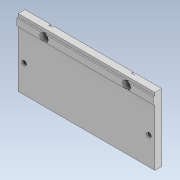
# Autodesk Inventor part: Klipper_Expander_Mount
Saved by Autodesk Inventor 2022.1 (Build 261234020, 234B)
## iProperties
Created: 2022-07-30
Part Number: Klipper_Expander_Mount
Material: Generisch
Document SubType Name: Modeling
Designer: Rama
Density: 1 g/cm^3
Appearance: Vorgabe
Author: Rama
Autodesk Inventor part; units mm, degrees
ref_plane "YZ Plane" through (0, 0, 0) normal (1, 0, 0) x (0, 1, 0)
ref_plane "XZ Plane" through (0, 0, 0) normal (0, 1, 0) x (-1, 0, 0)
ref_plane "XY Plane" through (0, 0, 0) normal (0, 0, 1) x (1, 0, 0)
sketch "Skizze1" plane through (0, 0, 0) normal (0, 0, 1) x (1, 0, 0)
  line L0 (50, -12) -> (-50, -12) projected
  line L1 (50, 12) -> (50, -12) projected
  line L2 (-50, 12) -> (50, 12) projected
  line L3 (-50, -12) -> (-50, 12) projected
  circle A0 centre (-21.494, -8.778) radius 0.5 projected
  circle A1 centre (-18.954, -8.778) radius 0.5 projected
  circle A2 centre (-13.874, -8.778) radius 0.5 projected
  circle A3 centre (-16.414, -8.778) radius 0.5 projected
  circle A4 centre (-3, 1.025) radius 0.85 projected
  circle A5 centre (-3, -2.635) radius 0.85 projected
  circle A6 centre (-1.67, -8.75) radius 0.5 projected
  circle A7 centre (-4.21, -8.75) radius 0.5 projected
  circle A8 centre (-6.75, -8.75) radius 0.5 projected
  circle A9 centre (-14.35, 5.5) radius 0.65 projected
  circle A10 centre (-9.27, 5.5) radius 0.65 projected
  circle A11 centre (-3, 5.495) radius 0.85 projected
  circle A12 centre (13.41, 5.5) radius 0.65 projected
  circle A13 centre (10.31, -9.613) radius 0.625 projected
  circle A14 centre (8.33, 5.5) radius 0.65 projected
  circle A15 centre (3.25, 5.5) radius 0.65 projected
  circle A16 centre (3.81, -9.613) radius 0.625 projected
  circle A17 centre (-26.341, -8.851) radius 0.5 projected
  circle A18 centre (-26.341, -6.311) radius 0.5 projected
  circle A19 centre (-26.341, -3.771) radius 0.5 projected
  circle A20 centre (-47.25, 1.58) radius 0.5 projected
  circle A21 centre (-47.25, -0.96) radius 0.5 projected
  circle A22 centre (-47.25, -3.5) radius 0.5 projected
  circle A23 centre (-41.75, -7.5) radius 0.5 projected
  circle A24 centre (-41.75, -4.96) radius 0.5 projected
  circle A25 centre (-47.25, -8.5) radius 0.5 projected
  circle A26 centre (-33, -4.96) radius 0.5 projected
  circle A27 centre (-33, -7.5) radius 0.5 projected
  circle A28 centre (-3, 9.155) radius 0.85 projected
  circle A29 centre (-34.242, 7.8785) radius 0.425 projected
  circle A30 centre (-29.242, 7.8785) radius 0.425 projected
  circle A31 centre (-22.54, 9) radius 0.5 projected
  circle A32 centre (-20, 9) radius 0.5 projected
  line L4 (-27.942, 10.9285) -> (-27.942, 10.2285) projected
  arc A33 (-28.542, 10.2285) -> (-27.942, 10.2285) centre (-28.242, 10.2285) ccw projected
  line L5 (-28.542, 10.2285) -> (-28.542, 10.9285) projected
  arc A34 (-27.942, 10.9285) -> (-28.542, 10.9285) centre (-28.242, 10.9285) ccw projected
  circle A35 centre (-46, 8) radius 1.6 projected
  line L6 (-34.942, 10.9285) -> (-34.942, 10.2285) projected
  arc A36 (-35.542, 10.2285) -> (-34.942, 10.2285) centre (-35.242, 10.2285) ccw projected
  line L7 (-35.542, 10.2285) -> (-35.542, 10.9285) projected
  arc A37 (-34.942, 10.9285) -> (-35.542, 10.9285) centre (-35.242, 10.9285) ccw projected
  circle A38 centre (33.73, 5.5) radius 0.65 projected
  circle A39 centre (28.65, 5.5) radius 0.65 projected
  circle A40 centre (18.49, 5.5) radius 0.65 projected
  circle A41 centre (23.57, 5.5) radius 0.65 projected
  circle A42 centre (38.81, 5.5) radius 0.65 projected
  circle A43 centre (46, 8) radius 1.6 projected
  line L8 (50.4, 12.4) -> (-50.4, 12.4)
  line L9 (-50.4, 12.4) -> (-50.4, -12.4)
  line L10 (-50.4, -12.4) -> (50.4, -12.4)
  line L11 (50.4, -12.4) -> (50.4, 12.4)
  point P0 (0, 0)
  dimension "d0" = 0.4
  dimension "d1" = 0.4
  dimension "d2" = 0.4
  dimension "d3" = 0.4
  constraints: 8 end point, 2 parallel, 1 horizontal, 1 perpendicular
  measures "d0" distance between parallel lines of L1 L11
  measures "d1" distance between parallel lines of L0 L10
  measures "d2" distance between parallel lines of L8 L2
  measures "d3" distance between parallel lines of L3 L9
extrude "Extrusion1" add sketch "Skizze1" along normal blind 6 contours L0 L3 L2 L1 | A0 | A1 | A2 | A3 | A4 | A5 | A6 | A7 | A8 | A9 | A10 | A11 | A12 | A13 | A14 | A15 | A16 | A17 | A18 | A19 | A20 | A21 | A22 | A23 | A24 | A25 | A26 | A27 | A28 | A29 | A30 | A31 | A32 | L4 A33 L5 A34 | A35 | L6 A36 L7 A37 | A38 | A39 | A40 | A41 | A42 | A43 | L11 L10 L9 L8
sketch "Skizze2" plane through (0, 0, 0) normal (0, 0, -1) x (-1, 0, 0)
  circle A0 centre (-46, 8) radius 1.6 projected
  circle A1 centre (46, 8) radius 1.6 projected
  point P0 (0, 0)
hole "Bohrung1" at (46, 8, 0) at (-46, 8, 0) direction (0, 0, 1) diameter 3.34 end through all counterbore diameter 4.7 counterbore depth 5
sketch "Skizze3" plane through (-50.4, 12.4, 0) normal (0, 1, 0) x (1, 0, 0)
  line L0 (100.8, 0) -> (0, 0) projected
  line L1 (0, 0) -> (0, -6) projected
  line L2 (100.8, -6) -> (0, -6) projected
  line L3 (100.8, 0) -> (100.8, -6) projected
  point P0 (50.4, 0)
extrude "Extrusion2" add sketch "Skizze3" along normal blind 25
sketch "Skizze4" plane through (50.4, -12.4, 6) normal (1, 0, 0) x (0, 0, -1)
  line L0 (0, 47.8) -> (-2, 47.8) projected
  line L1 (-2, 41.8) -> (0, 41.8) projected
  line L2 (7.6775, 47.7) -> (-1, 47.7)
  line L3 (-1, 47.7) -> (-1, 41.9)
  line L4 (-1, 41.9) -> (7.6775, 41.9)
  line L5 (7.6775, 41.9) -> (7.6775, 47.7)
  line L6 (0, 0) -> (0, 49.8) projected
  point P0 (6, 12.4)
  point P1 (0, 41.9)
  point P2 (0, 47.7)
  dimension "d15" = 0.1
  dimension "d16" = 0.1
  dimension "d17" = 5.8
  dimension "d18" = 1
  constraints: 8 end point, 2 parallel, 1 horizontal, 1 perpendicular
  measures "d15" distance between parallel lines of L0 L2
  measures "d16" distance between parallel lines of L1 L4
  measures "d17" distance of L4.end L2.start
  measures "d18" distance between parallel lines of L6 L3
extrude "Extrusion3" add sketch "Skizze4" against normal up to surface (100.8 mm away) contours L6 L4 L3 L2
sketch "Skizze6" plane through (0, 0, 0) normal (0, 0, -1) x (-1, 0, 0)
  line L0 (-50, -12) -> (50, -12) projected
  line L1 (-50, 12) -> (-50, -12) projected
  line L2 (50, 12) -> (-50, 12) projected
  line L3 (50, -12) -> (50, 12) projected
  circle A0 centre (21.494, -8.778) radius 0.5 projected
  circle A1 centre (18.954, -8.778) radius 0.5 projected
  circle A2 centre (13.874, -8.778) radius 0.5 projected
  circle A3 centre (16.414, -8.778) radius 0.5 projected
  circle A4 centre (3, 1.025) radius 0.85 projected
  circle A5 centre (3, -2.635) radius 0.85 projected
  circle A6 centre (1.67, -8.75) radius 0.5 projected
  circle A7 centre (4.21, -8.75) radius 0.5 projected
  circle A8 centre (6.75, -8.75) radius 0.5 projected
  circle A9 centre (14.35, 5.5) radius 0.65 projected
  circle A10 centre (9.27, 5.5) radius 0.65 projected
  circle A11 centre (3, 5.495) radius 0.85 projected
  circle A12 centre (-13.41, 5.5) radius 0.65 projected
  circle A13 centre (-10.31, -9.613) radius 0.625 projected
  circle A14 centre (-8.33, 5.5) radius 0.65 projected
  circle A15 centre (-3.25, 5.5) radius 0.65 projected
  circle A16 centre (-3.81, -9.613) radius 0.625 projected
  circle A17 centre (26.341, -8.851) radius 0.5 projected
  circle A18 centre (26.341, -6.311) radius 0.5 projected
  circle A19 centre (26.341, -3.771) radius 0.5 projected
  circle A20 centre (47.25, 1.58) radius 0.5 projected
  circle A21 centre (47.25, -0.96) radius 0.5 projected
  circle A22 centre (47.25, -3.5) radius 0.5 projected
  circle A23 centre (41.75, -7.5) radius 0.5 projected
  circle A24 centre (41.75, -4.96) radius 0.5 projected
  circle A25 centre (47.25, -8.5) radius 0.5 projected
  circle A26 centre (33, -4.96) radius 0.5 projected
  circle A27 centre (33, -7.5) radius 0.5 projected
  circle A28 centre (3, 9.155) radius 0.85 projected
  circle A29 centre (34.242, 7.8785) radius 0.425 projected
  circle A30 centre (29.242, 7.8785) radius 0.425 projected
  circle A31 centre (22.54, 9) radius 0.5 projected
  circle A32 centre (20, 9) radius 0.5 projected
  line L4 (27.942, 10.9285) -> (27.942, 10.2285) projected
  arc A33 (27.942, 10.2285) -> (28.542, 10.2285) centre (28.242, 10.2285) ccw projected
  line L5 (28.542, 10.2285) -> (28.542, 10.9285) projected
  arc A34 (28.542, 10.9285) -> (27.942, 10.9285) centre (28.242, 10.9285) ccw projected
  circle A35 centre (46, 8) radius 1.6 projected
  line L6 (34.942, 10.9285) -> (34.942, 10.2285) projected
  arc A36 (34.942, 10.2285) -> (35.542, 10.2285) centre (35.242, 10.2285) ccw projected
  line L7 (35.542, 10.2285) -> (35.542, 10.9285) projected
  arc A37 (35.542, 10.9285) -> (34.942, 10.9285) centre (35.242, 10.9285) ccw projected
  circle A38 centre (-33.73, 5.5) radius 0.65 projected
  circle A39 centre (-28.65, 5.5) radius 0.65 projected
  circle A40 centre (-18.49, 5.5) radius 0.65 projected
  circle A41 centre (-23.57, 5.5) radius 0.65 projected
  circle A42 centre (-38.81, 5.5) radius 0.65 projected
  circle A43 centre (-46, 8) radius 1.6 projected
  point P0 (0, 0)
hole "Bohrung2" at (38.81, 5.5, 0) at (33.73, 5.5, 0) at (28.65, 5.5, 0) at (23.57, 5.5, 0) at (18.49, 5.5, 0) at (13.41, 5.5, 0) at (8.33, 5.5, 0) at (3.25, 5.5, 0) at (-3, 5.495, 0) at (-3, 9.155, 0) at (-3, 1.025, 0) at (-3, -2.635, 0) at (-9.27, 5.5, 0) at (-14.35, 5.5, 0) direction (0, 0, 1) diameter 2.8 depth 2 tip angle 60
sketch "Skizze7" plane through (0, 0, 0) normal (0, 0, -1) x (-1, 0, 0)
  line L0 (-50, -12) -> (50, -12) projected
  line L1 (-50, 12) -> (-50, -12) projected
  line L2 (50, 12) -> (-50, 12) projected
  line L3 (50, -12) -> (50, 12) projected
  circle A0 centre (21.494, -8.778) radius 0.5 projected
  circle A1 centre (18.954, -8.778) radius 0.5 projected
  circle A2 centre (13.874, -8.778) radius 0.5 projected
  circle A3 centre (16.414, -8.778) radius 0.5 projected
  circle A4 centre (3, 1.025) radius 0.85 projected
  circle A5 centre (3, -2.635) radius 0.85 projected
  circle A6 centre (1.67, -8.75) radius 0.5 projected
  circle A7 centre (4.21, -8.75) radius 0.5 projected
  circle A8 centre (6.75, -8.75) radius 0.5 projected
  circle A9 centre (14.35, 5.5) radius 0.65 projected
  circle A10 centre (9.27, 5.5) radius 0.65 projected
  circle A11 centre (3, 5.495) radius 0.85 projected
  circle A12 centre (-13.41, 5.5) radius 0.65 projected
  circle A13 centre (-10.31, -9.613) radius 0.625 projected
  circle A14 centre (-8.33, 5.5) radius 0.65 projected
  circle A15 centre (-3.25, 5.5) radius 0.65 projected
  circle A16 centre (-3.81, -9.613) radius 0.625 projected
  circle A17 centre (26.341, -8.851) radius 0.5 projected
  circle A18 centre (26.341, -6.311) radius 0.5 projected
  circle A19 centre (26.341, -3.771) radius 0.5 projected
  circle A20 centre (47.25, 1.58) radius 0.5 projected
  circle A21 centre (47.25, -0.96) radius 0.5 projected
  circle A22 centre (47.25, -3.5) radius 0.5 projected
  circle A23 centre (41.75, -7.5) radius 0.5 projected
  circle A24 centre (41.75, -4.96) radius 0.5 projected
  circle A25 centre (47.25, -8.5) radius 0.5 projected
  circle A26 centre (33, -4.96) radius 0.5 projected
  circle A27 centre (33, -7.5) radius 0.5 projected
  circle A28 centre (3, 9.155) radius 0.85 projected
  circle A29 centre (34.242, 7.8785) radius 0.425 projected
  circle A30 centre (29.242, 7.8785) radius 0.425 projected
  circle A31 centre (22.54, 9) radius 0.5 projected
  circle A32 centre (20, 9) radius 0.5 projected
  line L4 (27.942, 10.9285) -> (27.942, 10.2285) projected
  arc A33 (27.942, 10.2285) -> (28.542, 10.2285) centre (28.242, 10.2285) ccw projected
  line L5 (28.542, 10.2285) -> (28.542, 10.9285) projected
  arc A34 (28.542, 10.9285) -> (27.942, 10.9285) centre (28.242, 10.9285) ccw projected
  circle A35 centre (46, 8) radius 1.6 projected
  line L6 (34.942, 10.9285) -> (34.942, 10.2285) projected
  arc A36 (34.942, 10.2285) -> (35.542, 10.2285) centre (35.242, 10.2285) ccw projected
  line L7 (35.542, 10.2285) -> (35.542, 10.9285) projected
  arc A37 (35.542, 10.9285) -> (34.942, 10.9285) centre (35.242, 10.9285) ccw projected
  circle A38 centre (-33.73, 5.5) radius 0.65 projected
  circle A39 centre (-28.65, 5.5) radius 0.65 projected
  circle A40 centre (-18.49, 5.5) radius 0.65 projected
  circle A41 centre (-23.57, 5.5) radius 0.65 projected
  circle A42 centre (-38.81, 5.5) radius 0.65 projected
  circle A43 centre (-46, 8) radius 1.6 projected
  point P0 (0, 0)
hole "Bohrung3" at (10.31, -9.613, 0) at (3.81, -9.613, 0) at (-1.67, -8.75, 0) at (-4.21, -8.75, 0) at (-6.75, -8.75, 0) at (-13.874, -8.778, 0) at (-16.414, -8.778, 0) at (-18.954, -8.778, 0) at (-21.494, -8.778, 0) at (-26.341, -8.851, 0) at (-26.341, -6.311, 0) at (-26.341, -3.771, 0) at (-47.25, -8.5, 0) at (-47.25, -3.5, 0) at (-47.25, -0.96, 0) at (-47.25, 1.58, 0) at (-22.54, 9, 0) at (-20, 9, 0) direction (0, 0, 1) diameter 2 depth 1.4 tip angle 60
sketch "Skizze8" plane through (0, 0, 0) normal (0, 0, -1) x (-1, 0, 0)
  line L0 (-50, -12) -> (50, -12) projected
  line L1 (-50, 12) -> (-50, -12) projected
  line L2 (50, 12) -> (-50, 12) projected
  line L3 (50, -12) -> (50, 12) projected
  circle A0 centre (21.494, -8.778) radius 0.5 projected
  circle A1 centre (18.954, -8.778) radius 0.5 projected
  circle A2 centre (13.874, -8.778) radius 0.5 projected
  circle A3 centre (16.414, -8.778) radius 0.5 projected
  circle A4 centre (3, 1.025) radius 0.85 projected
  circle A5 centre (3, -2.635) radius 0.85 projected
  circle A6 centre (1.67, -8.75) radius 0.5 projected
  circle A7 centre (4.21, -8.75) radius 0.5 projected
  circle A8 centre (6.75, -8.75) radius 0.5 projected
  circle A9 centre (14.35, 5.5) radius 0.65 projected
  circle A10 centre (9.27, 5.5) radius 0.65 projected
  circle A11 centre (3, 5.495) radius 0.85 projected
  circle A12 centre (-13.41, 5.5) radius 0.65 projected
  circle A13 centre (-10.31, -9.613) radius 0.625 projected
  circle A14 centre (-8.33, 5.5) radius 0.65 projected
  circle A15 centre (-3.25, 5.5) radius 0.65 projected
  circle A16 centre (-3.81, -9.613) radius 0.625 projected
  circle A17 centre (26.341, -8.851) radius 0.5 projected
  circle A18 centre (26.341, -6.311) radius 0.5 projected
  circle A19 centre (26.341, -3.771) radius 0.5 projected
  circle A20 centre (47.25, 1.58) radius 0.5 projected
  circle A21 centre (47.25, -0.96) radius 0.5 projected
  circle A22 centre (47.25, -3.5) radius 0.5 projected
  circle A23 centre (41.75, -7.5) radius 0.5 projected
  circle A24 centre (41.75, -4.96) radius 0.5 projected
  circle A25 centre (47.25, -8.5) radius 0.5 projected
  circle A26 centre (33, -4.96) radius 0.5 projected
  circle A27 centre (33, -7.5) radius 0.5 projected
  circle A28 centre (3, 9.155) radius 0.85 projected
  circle A29 centre (34.242, 7.8785) radius 0.425 projected
  circle A30 centre (29.242, 7.8785) radius 0.425 projected
  circle A31 centre (22.54, 9) radius 0.5 projected
  circle A32 centre (20, 9) radius 0.5 projected
  line L4 (27.942, 10.9285) -> (27.942, 10.2285) projected
  arc A33 (27.942, 10.2285) -> (28.542, 10.2285) centre (28.242, 10.2285) ccw projected
  line L5 (28.542, 10.2285) -> (28.542, 10.9285) projected
  arc A34 (28.542, 10.9285) -> (27.942, 10.9285) centre (28.242, 10.9285) ccw projected
  circle A35 centre (46, 8) radius 1.6 projected
  line L6 (34.942, 10.9285) -> (34.942, 10.2285) projected
  arc A36 (34.942, 10.2285) -> (35.542, 10.2285) centre (35.242, 10.2285) ccw projected
  line L7 (35.542, 10.2285) -> (35.542, 10.9285) projected
  arc A37 (35.542, 10.9285) -> (34.942, 10.9285) centre (35.242, 10.9285) ccw projected
  circle A38 centre (-33.73, 5.5) radius 0.65 projected
  circle A39 centre (-28.65, 5.5) radius 0.65 projected
  circle A40 centre (-18.49, 5.5) radius 0.65 projected
  circle A41 centre (-23.57, 5.5) radius 0.65 projected
  circle A42 centre (-38.81, 5.5) radius 0.65 projected
  circle A43 centre (-46, 8) radius 1.6 projected
  line L8 (30.641, -7.5) -> (33.181, -7.5)
  line L9 (33.181, -7.5) -> (33.181, -9.351)
  line L10 (33.181, -9.351) -> (30.641, -9.351)
  line L11 (30.641, -9.351) -> (30.641, -7.5)
  line L12 (39.331, -7.5) -> (41.871, -7.5)
  line L13 (41.871, -7.5) -> (41.871, -9.613)
  line L14 (41.871, -9.613) -> (39.331, -9.613)
  line L15 (39.331, -9.613) -> (39.331, -7.5)
  point P0 (0, 0)
  dimension "d36" = 2.54
  dimension "d37" = 6.659
  dimension "d38" = 8.75
  dimension "d39" = 2.54
  dimension "d40" = 2.54
  dimension "d41" = 6.15
  dimension "d42" = 4.3
  dimension "d43" = 5.379
  constraints: 16 end point, 4 parallel, 2 horizontal, 2 perpendicular, 2 point on line
  measures "d36" distance of A27.centre A26.centre
  measures "d37" horizontal distance of A27.centre A18.centre
  measures "d38" distance of A23.centre A27.centre
  measures "d39" distance of L9.end L10.end
  measures "d40" distance of L13.end L14.end
  measures "d41" distance between parallel lines of L15 L9
  measures "d42" distance from line of L11 A17.centre
  measures "d43" distance from line of L13 A25.centre
hole "Bohrung4" at (-33.181, -7.5, 0) at (-30.641, -7.5, 0) at (-39.331, -7.5, 0) at (-41.871, -7.5, 0) direction (0, 0, 1) diameter 2 depth 1.4 tip angle 60
sketch "Skizze9" plane through (0, 0, 0) normal (0, 0, -1) x (-1, 0, 0)
  line L0 (-50.4, 29.5) -> (50.4, 29.5) projected
  line L1 (50.4, 35.3) -> (-50.4, 35.3) projected
  line L2 (50.4, 37.4) -> (50.4, -12.4) projected
  line L3 (-50.4, -12.4) -> (-50.4, 37.4) projected
  point P0 (0, 0)
  point P1 (-30.4, 32.4)
  point P2 (30.4, 32.4)
  dimension "d51" = 5.8
  dimension "d52" = 2.9
  dimension "d53" = 2.9
  dimension "d54" = 20
  dimension "d55" = 20
  measures "d51" distance between parallel lines of L0 L1
  measures "d52" distance from line of point (-30.4, 32.4) L0
  measures "d53" distance from line of point (30.4, 32.4) L0
  measures "d54" distance from line of L2 point (30.4, 32.4)
  measures "d55" distance from line of L3 point (-30.4, 32.4)
hole "Bohrung5" at (-30.4, 32.4, 0) at (30.4, 32.4, 0) direction (0, 0, 1) diameter 5.4 end through all counterbore diameter 9.4 counterbore depth 2.8
chamfer "Fase1" distance 1 angle 45 4 edges at (0, 37.4, 0) (50.4, 12.5, 0) (-50.4, 12.5, 0) (0, -12.4, 0)
chamfer "Fase2" distance 0.4 angle 45 16 edges at (46, 5.65, 0) (38.81, 4.1, 0) (33.73, 4.1, 0) (28.65, 4.1, 0) (23.57, 4.1, 0) (18.49, 4.1, 0) (13.41, 4.1, 0) (8.33, 4.1, 0) (3.25, 4.1, 0) (-3, 7.755, 0) (-3, 4.095, 0) (-3, -0.375, 0) (-3, -4.035, 0) (-9.27, 4.1, 0) (-14.35, 4.1, 0) (-46, 5.65, 0)
sketch "Skizze10" plane through (0, 0, 0) normal (0, 0, -1) x (-1, 0, 0)
  circle A0 centre (14.35, 5.5) radius 1.8 projected
  circle A1 centre (3, -2.635) radius 1.8 projected
  circle A2 centre (3, 5.495) radius 1.8 projected
  circle A3 centre (-3.25, 5.5) radius 1.8 projected
  circle A4 centre (-13.41, 5.5) radius 1.8 projected
  circle A5 centre (-23.57, 5.5) radius 1.8 projected
  circle A6 centre (-33.73, 5.5) radius 1.8 projected
  circle A7 centre (-46, 8) radius 2.75 projected
  line L0 (32.8678, 36.4) -> (49.4, 36.4) projected
  arc A8 (27.9322, 36.4) -> (32.8678, 36.4) centre (30.4, 32.4) ccw projected
  line L1 (-27.9322, 36.4) -> (27.9322, 36.4) projected
  arc A9 (-32.8678, 36.4) -> (-27.9322, 36.4) centre (-30.4, 32.4) ccw projected
  line L2 (-49.4, 36.4) -> (-32.8678, 36.4) projected
  line L3 (-49.4, -11.4) -> (-49.4, 36.4) projected
  line L4 (49.4, -11.4) -> (-49.4, -11.4) projected
  line L5 (49.4, 36.4) -> (49.4, -11.4) projected
  circle A10 centre (39.331, -7.5) radius 1 projected
  circle A11 centre (33.181, -7.5) radius 1 projected
  circle A12 centre (30.641, -7.5) radius 1 projected
  circle A13 centre (41.871, -7.5) radius 1 projected
  circle A14 centre (22.54, 9) radius 1 projected
  circle A15 centre (47.25, -0.96) radius 1 projected
  circle A16 centre (47.25, -8.5) radius 1 projected
  circle A17 centre (26.341, -6.311) radius 1 projected
  circle A18 centre (21.494, -8.778) radius 1 projected
  circle A19 centre (16.414, -8.778) radius 1 projected
  circle A20 centre (6.75, -8.75) radius 1 projected
  circle A21 centre (1.67, -8.75) radius 1 projected
  circle A22 centre (-10.31, -9.613) radius 1 projected
  circle A23 centre (-3.81, -9.613) radius 1 projected
  circle A24 centre (4.21, -8.75) radius 1 projected
  circle A25 centre (13.874, -8.778) radius 1 projected
  circle A26 centre (18.954, -8.778) radius 1 projected
  circle A27 centre (26.341, -8.851) radius 1 projected
  circle A28 centre (26.341, -3.771) radius 1 projected
  circle A29 centre (47.25, -3.5) radius 1 projected
  circle A30 centre (47.25, 1.58) radius 1 projected
  circle A31 centre (20, 9) radius 1 projected
  circle A32 centre (-38.81, 5.5) radius 1.8 projected
  circle A33 centre (-28.65, 5.5) radius 1.8 projected
  circle A34 centre (-18.49, 5.5) radius 1.8 projected
  circle A35 centre (-8.33, 5.5) radius 1.8 projected
  circle A36 centre (3, 9.155) radius 1.8 projected
  circle A37 centre (3, 1.025) radius 1.8 projected
  circle A38 centre (9.27, 5.5) radius 1.8 projected
  circle A39 centre (46, 8) radius 2.75 projected
  line L6 (-31.4, 39.3857) -> (-29.4, 39.3857)
  line L7 (-29.4, 39.3857) -> (-29.4, 35.7506)
  line L8 (-29.4, 35.7506) -> (-31.4, 35.7506)
  line L9 (-31.4, 35.7506) -> (-31.4, 39.3857)
  line L10 (29.4, 38.7324) -> (31.4, 38.7324)
  line L11 (31.4, 38.7324) -> (31.4, 35.5237)
  line L12 (31.4, 35.5237) -> (29.4, 35.5237)
  line L13 (29.4, 35.5237) -> (29.4, 38.7324)
  point P0 (0, 0)
  point P1 (-30.4, 35.7506)
  point P2 (30.4, 35.5237)
  dimension "d69" = 0
  dimension "d70" = 0
  dimension "d71" = 2
  dimension "d72" = 2
  constraints: 16 end point, 4 parallel, 2 horizontal, 2 midpoint, 2 perpendicular
  measures "d69" horizontal distance of A9.centre point (-30.4, 35.751)
  measures "d70" horizontal distance of A8.centre point (30.4, 35.524)
  measures "d71" distance of L6.start L6.end
  measures "d72" distance of L10.start L10.end
extrude "Extrusion4" cut sketch "Skizze10" against normal up to surface (2.8 mm away) contours L6 L7 L8 L9 | L10 L11 L12 L13
sketch "Skizze11" plane through (30.4, 32.4, 2.8) normal (0, 0, -1) x (-1, 0, 0)
  circle A0 centre (0, 0) radius 2.7 projected
  arc A1 (-1, 4.5924) -> (1, 4.5924) centre (0, 0) ccw projected
  line L0 (1, 4.5924) -> (1, 5) projected
  line L1 (-1, 5) -> (1, 5) projected
  line L2 (-1, 5) -> (-1, 4.5924) projected
  arc A2 (59.8, 4.5924) -> (61.8, 4.5924) centre (60.8, 0) ccw projected
  line L3 (61.8, 4.5924) -> (61.8, 5) projected
  line L4 (59.8, 5) -> (61.8, 5) projected
  line L5 (59.8, 5) -> (59.8, 4.5924) projected
  circle A3 centre (60.8, 0) radius 2.7 projected
  line L6 (-2.7, 8.7587) -> (2.7, 8.7587)
  line L7 (2.7, 8.7587) -> (2.7, -10.1015)
  line L8 (2.7, -10.1015) -> (-2.7, -10.1015)
  line L9 (-2.7, -10.1015) -> (-2.7, 8.7587)
  line L10 (58.1, 8.7587) -> (63.5, 8.7587)
  line L11 (63.5, 8.7587) -> (63.5, -8.4106)
  line L12 (63.5, -8.4106) -> (58.1, -8.4106)
  line L13 (58.1, -8.4106) -> (58.1, 8.7587)
  circle A4 centre (0, 0) radius 2.7 projected
  circle A5 centre (60.8, 0) radius 2.7 projected
  point P0 (30.4, -32.4)
  point P1 (63.5, -3.8471)
  point P2 (63.5, 3.8471)
  point P3 (58.1, 3.8471)
  point P4 (58.1, -3.8471)
  point P5 (2.7, -3.8471)
  point P6 (2.7, 3.8471)
  point P7 (-2.7, 3.8471)
  point P8 (-2.7, -3.8471)
  constraints: 16 end point, 4 parallel, 4 tangent, 2 horizontal, 2 perpendicular, 1 point on line
extrude "Extrusion5" add sketch "Skizze11" along normal blind 0.2 contours L7 A1 | L9 A1 | L13 A2 | L11 A2
sketch "Skizze12" plane through (30.4, 32.4, 2.8) normal (0, 0, -1) x (-1, 0, 0)
  line L0 (2.7, -3.8471) -> (2.7, 0) projected
  arc A0 (-2.7, 0) -> (2.7, 0) centre (0, 0) ccw projected
  line L1 (-2.7, 0) -> (-2.7, -3.8471) projected
  arc A1 (-2.7, -3.8471) -> (2.7, -3.8471) centre (0, 0) ccw projected
  arc A2 (63.5, 0) -> (58.1, 0) centre (60.8, 0) ccw projected
  arc A3 (58.3322, 4) -> (63.2678, 4) centre (60.8, 0) ccw projected
  arc A4 (-2.4678, 4) -> (2.4678, 4) centre (0, 0) ccw projected
  arc A5 (2.7, 0) -> (-2.7, 0) centre (0, 0) ccw projected
  arc A6 (58.1, 0) -> (63.5, 0) centre (60.8, 0) ccw projected
  arc A7 (2.4678, 4) -> (1, 4.5924) centre (0, 0) ccw projected
  arc A8 (-1, 4.5924) -> (-2.4678, 4) centre (0, 0) ccw projected
  line L2 (2.7, 0) -> (2.7, 3.8471) projected
  arc A9 (2.7, 3.8471) -> (1, 4.5924) centre (0, 0) ccw projected
  line L3 (1, 4.5924) -> (1, 5) projected
  line L4 (-1, 5) -> (1, 5) projected
  line L5 (-1, 5) -> (-1, 4.5924) projected
  arc A10 (-1, 4.5924) -> (-2.7, 3.8471) centre (0, 0) ccw projected
  line L6 (-2.7, 3.8471) -> (-2.7, 0) projected
  arc A11 (2.7, 0) -> (-2.7, 0) centre (0, 0) ccw projected
  line L7 (58.1, 3.8471) -> (58.1, 0) projected
  arc A12 (63.5, 0) -> (58.1, 0) centre (60.8, 0) ccw projected
  line L8 (63.5, 0) -> (63.5, 3.8471) projected
  arc A13 (63.5, 3.8471) -> (61.8, 4.5924) centre (60.8, 0) ccw projected
  line L9 (61.8, 4.5924) -> (61.8, 5) projected
  line L10 (59.8, 5) -> (61.8, 5) projected
  line L11 (59.8, 5) -> (59.8, 4.5924) projected
  arc A14 (59.8, 4.5924) -> (58.1, 3.8471) centre (60.8, 0) ccw projected
  line L12 (-10.6112, -2.7) -> (72.9159, -2.7)
  line L13 (72.9159, -2.7) -> (72.9159, 2.7)
  line L14 (72.9159, 2.7) -> (-10.6112, 2.7)
  line L15 (-10.6112, 2.7) -> (-10.6112, -2.7)
  arc A15 (-2.7, 0) -> (2.7, 0) centre (0, 0) ccw projected
  circle A16 centre (44.75, -26.9) radius 1.8 projected
  circle A17 centre (33.4, -35.035) radius 1.8 projected
  circle A18 centre (33.4, -26.905) radius 1.8 projected
  circle A19 centre (27.15, -26.9) radius 1.8 projected
  circle A20 centre (16.99, -26.9) radius 1.8 projected
  circle A21 centre (6.83, -26.9) radius 1.8 projected
  circle A22 centre (-3.33, -26.9) radius 1.8 projected
  circle A23 centre (-15.6, -24.4) radius 2.75 projected
  line L16 (63.2678, 4) -> (79.8, 4) projected
  arc A24 (58.3322, 4) -> (63.2678, 4) centre (60.8, 0) ccw projected
  line L17 (2.4678, 4) -> (58.3322, 4) projected
  arc A25 (-2.4678, 4) -> (2.4678, 4) centre (0, 0) ccw projected
  line L18 (-19, 4) -> (-2.4678, 4) projected
  line L19 (-19, -43.8) -> (-19, 4) projected
  line L20 (79.8, -43.8) -> (-19, -43.8) projected
  line L21 (79.8, 4) -> (79.8, -43.8) projected
  circle A26 centre (69.731, -39.9) radius 1 projected
  circle A27 centre (63.581, -39.9) radius 1 projected
  circle A28 centre (61.041, -39.9) radius 1 projected
  circle A29 centre (72.271, -39.9) radius 1 projected
  circle A30 centre (52.94, -23.4) radius 1 projected
  circle A31 centre (77.65, -33.36) radius 1 projected
  circle A32 centre (77.65, -40.9) radius 1 projected
  circle A33 centre (56.741, -38.711) radius 1 projected
  circle A34 centre (51.894, -41.178) radius 1 projected
  circle A35 centre (46.814, -41.178) radius 1 projected
  circle A36 centre (37.15, -41.15) radius 1 projected
  circle A37 centre (32.07, -41.15) radius 1 projected
  circle A38 centre (20.09, -42.013) radius 1 projected
  circle A39 centre (26.59, -42.013) radius 1 projected
  circle A40 centre (34.61, -41.15) radius 1 projected
  circle A41 centre (44.274, -41.178) radius 1 projected
  circle A42 centre (49.354, -41.178) radius 1 projected
  circle A43 centre (56.741, -41.251) radius 1 projected
  circle A44 centre (56.741, -36.171) radius 1 projected
  circle A45 centre (77.65, -35.9) radius 1 projected
  circle A46 centre (77.65, -30.82) radius 1 projected
  circle A47 centre (50.4, -23.4) radius 1 projected
  circle A48 centre (-8.41, -26.9) radius 1.8 projected
  circle A49 centre (1.75, -26.9) radius 1.8 projected
  circle A50 centre (11.91, -26.9) radius 1.8 projected
  circle A51 centre (22.07, -26.9) radius 1.8 projected
  circle A52 centre (33.4, -23.245) radius 1.8 projected
  circle A53 centre (33.4, -31.375) radius 1.8 projected
  circle A54 centre (39.67, -26.9) radius 1.8 projected
  circle A55 centre (76.4, -24.4) radius 2.75 projected
  point P0 (30.4, -32.4)
  point P1 (64.6471, -2.7)
  point P2 (56.9529, -2.7)
  point P3 (56.9529, 2.7)
  point P4 (64.6471, 2.7)
  point P5 (-3.8471, 2.7)
  point P6 (3.8471, 2.7)
  point P7 (-3.8471, -2.7)
  point P8 (3.8471, -2.7)
  constraints: 8 end point, 2 parallel, 2 tangent, 1 horizontal, 1 perpendicular
extrude "Extrusion6" add sketch "Skizze12" along normal blind 0.4 contours A1 L1 L12 L0 | L0 L12 A4 | A4 L12 L1 | L14 L2 A4 | L12 A3 | L14 L6 A4 A8 L5 L4 L3 A7 L2 | A4 L6 L14 | A3 L7 L14 | A3 A14 L11 L10 L9 A13 L8 L14 L7 | L14 L8 A3
sketch "Skizze13" plane through (50.4, 29.5, 7) normal (0, 0, 1) x (1, 0, 0)
  circle A0 centre (-80.8, 2.9) radius 2.7 projected
  circle A1 centre (-80.8, 2.9) radius 2.7 projected
  circle A2 centre (-20, 2.9) radius 2.7 projected
  line L0 (-100.8, 5.8) -> (-100.8, 0) projected
  line L1 (0, 0) -> (-100.8, 0) projected
  line L2 (0, 5.8) -> (0, 0) projected
  line L3 (0, 5.8) -> (-100.8, 5.8) projected
  line L4 (-81.6, 10.5152) -> (-80, 10.5152)
  line L5 (-80, 10.5152) -> (-80, -5.0723)
  line L6 (-80, -5.0723) -> (-81.6, -5.0723)
  line L7 (-81.6, -5.0723) -> (-81.6, 10.5152)
  line L8 (-20.8, 13.9368) -> (-19.2, 13.9368)
  line L9 (-19.2, 13.9368) -> (-19.2, -6.5931)
  line L10 (-19.2, -6.5931) -> (-20.8, -6.5931)
  line L11 (-20.8, -6.5931) -> (-20.8, 13.9368)
  point P0 (-50.4, -29.5)
  point P1 (-80.8, -5.0723)
  point P2 (-20, -6.5931)
  dimension "d79" = 0
  dimension "d80" = 0
  dimension "d81" = 1.6
  dimension "d82" = 1.6
  constraints: 16 end point, 4 parallel, 2 horizontal, 2 midpoint, 2 perpendicular
  measures "d79" horizontal distance of A0.centre point (-80.8, -5.072)
  measures "d80" horizontal distance of point (-20, -6.593) A2.centre
  measures "d81" distance of L5.end L6.end
  measures "d82" distance of L9.end L10.end
extrude "Extrusion7" cut sketch "Skizze13" against normal up to surface (1 mm away) contours L5 A0 L7 | A0 L7 L3 L5 | L5 L1 L7 A0 | L3 L7 L4 L5 | L5 L6 L7 L1 | L11 L8 L9 L3 | L3 L9 A2 L11 | L11 A2 L9 L1 | L1 L9 L10 L11 | A2 L9 L11
chamfer "Fase3" distance 0.4 angle 45 10 edges at (0, 35.3, 7) (0, 29.5, 7) (-40.8, 29.5, 7) (-40.8, 35.3, 7) (-33.1, 32.4, 7) (-27.7, 32.4, 7) (27.7, 32.4, 7) (33.1, 32.4, 7) (40.8, 35.3, 7) (40.8, 29.5, 7)
sketch "Skizze14" plane through (0, 0, 0) normal (0, 0, -1) x (-1, 0, 0)
  line L0 (-41.35, 3.5906) -> (-41.35, 7.7829) projected
  line L1 (-0.71, 7.7829) -> (-41.35, 7.7829) projected
  line L2 (-41.35, 3.5906) -> (-41.35, 7.7829) projected
  line L3 (-41.35, 3.5906) -> (-0.71, 3.5906) projected
  line L4 (-0.71, 7.7829) -> (-0.71, 3.5906) projected
  circle A0 centre (-26.11, 4.4) radius 0.4899 projected
  circle A1 centre (-13.41, 5.7) radius 2 projected
  circle A2 centre (-15.95, 4.4) radius 0.4899 projected
  circle A3 centre (-5.79, 4.4) radius 0.4899 projected
  circle A4 centre (-3.25, 5.7) radius 2 projected
  circle A5 centre (-10.87, 4.4) radius 0.4899 projected
  circle A6 centre (-8.33, 5.7) radius 2 projected
  circle A7 centre (-18.49, 5.7) radius 2 projected
  circle A8 centre (-21.03, 4.4) radius 0.4899 projected
  circle A9 centre (-23.57, 5.7) radius 2 projected
  circle A10 centre (-31.19, 4.4) radius 0.4899 projected
  circle A11 centre (-28.65, 5.7) radius 2 projected
  circle A12 centre (-36.27, 4.4) radius 0.4899 projected
  circle A13 centre (-33.73, 5.7) radius 2 projected
  circle A14 centre (-38.81, 5.7) radius 2 projected
  line L5 (16.89, 7.7829) -> (6.73, 7.7829) projected
  line L6 (6.73, 3.5906) -> (6.73, 7.7829) projected
  line L7 (6.73, 3.5906) -> (16.89, 3.5906) projected
  line L8 (16.89, 7.7829) -> (16.89, 3.5906) projected
  circle A15 centre (11.81, 4.4) radius 0.4899 projected
  circle A16 centre (14.35, 5.7) radius 2 projected
  circle A17 centre (9.27, 5.7) radius 2 projected
  line L9 (-51.35, 17.7829) -> (9.29, 17.7829) construction
  line L10 (9.29, 17.7829) -> (9.29, 11.7829) construction
  line L11 (9.29, 11.7829) -> (-51.35, 11.7829) construction
  line L12 (-51.35, 11.7829) -> (-51.35, 17.7829) construction
  line L13 (6.73, 17.7829) -> (16.89, 17.7829) construction
  line L14 (16.89, 17.7829) -> (16.89, 11.7829) construction
  line L15 (16.89, 11.7829) -> (6.73, 11.7829) construction
  line L16 (6.73, 11.7829) -> (6.73, 17.7829) construction
  line L17 (-38.4318, 14.1885) -> (-38.8845, 14.1885)
  line L18 (-38.8845, 14.1885) -> (-38.8845, 12.8829)
  line L19 (-38.8845, 12.8829) -> (-39.3741, 12.8829)
  line L20 (-39.3741, 12.8829) -> (-39.3741, 14.1885)
  line L21 (-39.3741, 14.1885) -> (-41.0524, 14.1885)
  line L22 (-41.0524, 14.1885) -> (-41.0524, 14.7244)
  line L23 (-41.0524, 14.7244) -> (-39.3525, 16.6829)
  line L24 (-39.3525, 16.6829) -> (-38.8845, 16.6829)
  line L25 (-38.8845, 16.6829) -> (-38.8845, 14.5981)
  line L26 (-38.8845, 14.5981) -> (-38.4318, 14.5981)
  line L27 (-38.4318, 14.5981) -> (-38.4318, 14.1885)
  line L28 (-39.3741, 14.5981) -> (-39.3741, 16.0824)
  line L29 (-39.3741, 16.0824) -> (-40.652, 14.5981)
  line L30 (-40.652, 14.5981) -> (-39.3741, 14.5981)
  line L31 (-33.5294, 16.6829) -> (-34.8381, 12.8829)
  line L32 (-34.8381, 12.8829) -> (-35.3832, 12.8829)
  line L33 (-35.3832, 12.8829) -> (-36.6919, 16.6829)
  line L34 (-36.6919, 16.6829) -> (-36.1499, 16.6829)
  line L35 (-36.1499, 16.6829) -> (-35.0968, 13.5265)
  line L36 (-35.0968, 13.5265) -> (-34.0436, 16.6829)
  line L37 (-34.0436, 16.6829) -> (-33.5294, 16.6829)
  spline S0 degree 2 poles (-28.9841, 16.3226) (-29.1227, 16.3226) (-29.3968, 16.2548) (-29.5292, 16.2025) knots 0 0 0 1 2 2 2
  spline S1 degree 2 poles (-29.5292, 16.2025) (-29.6524, 16.1501) (-29.8341, 16.0393) (-29.9049, 15.99) knots 0 0 0 1 2 2 2
  line L38 (-29.9049, 15.99) -> (-29.9357, 15.99)
  line L39 (-29.9357, 15.99) -> (-29.9357, 16.5289)
  spline S2 degree 2 poles (-29.9357, 16.5289) (-29.7694, 16.6182) (-29.1997, 16.7629) (-28.9441, 16.7629) knots 0 0 0 1 2 2 2
  spline S3 degree 2 poles (-28.9441, 16.7629) (-28.6854, 16.7629) (-28.3005, 16.6582) (-28.1435, 16.5474) knots 0 0 0 1 2 2 2
  spline S4 degree 2 poles (-28.1435, 16.5474) (-27.9772, 16.4273) (-27.8047, 16.0793) (-27.8047, 15.8453) knots 0 0 0 1 2 2 2
  spline S5 degree 2 poles (-27.8047, 15.8453) (-27.8047, 15.5312) (-28.2174, 15.0569) (-28.5068, 14.9953) knots 0 0 0 1 2 2 2
  line L40 (-28.5068, 14.9953) -> (-28.5068, 14.9584)
  spline S6 degree 2 poles (-28.5068, 14.9584) (-28.3867, 14.9338) (-28.1127, 14.8229) (-27.9956, 14.712) knots 0 0 0 1 2 2 2
  spline S7 degree 2 poles (-27.9956, 14.712) (-27.8786, 14.6043) (-27.7308, 14.2594) (-27.7308, 14.0099) knots 0 0 0 1 2 2 2
  spline S8 degree 2 poles (-27.7308, 14.0099) (-27.7308, 13.7543) (-27.9063, 13.3201) (-28.0665, 13.1539) knots 0 0 0 1 2 2 2
  spline S9 degree 2 poles (-28.0665, 13.1539) (-28.2328, 12.9814) (-28.7039, 12.8028) (-29.0026, 12.8028) knots 0 0 0 1 2 2 2
  spline S10 degree 2 poles (-29.0026, 12.8028) (-29.289, 12.8028) (-29.8494, 12.9414) (-30.0404, 13.0368) knots 0 0 0 1 2 2 2
  line L41 (-30.0404, 13.0368) -> (-30.0404, 13.5757)
  line L42 (-30.0404, 13.5757) -> (-30.0034, 13.5757)
  spline S11 degree 2 poles (-30.0034, 13.5757) (-29.8433, 13.4587) (-29.3013, 13.2432) (-29.0334, 13.2432) knots 0 0 0 1 2 2 2
  spline S12 degree 2 poles (-29.0334, 13.2432) (-28.8764, 13.2432) (-28.5623, 13.3417) (-28.4576, 13.4556) knots 0 0 0 1 2 2 2
  spline S13 degree 2 poles (-28.4576, 13.4556) (-28.3559, 13.5696) (-28.2482, 13.8406) (-28.2482, 14.0469) knots 0 0 0 1 2 2 2
  spline S14 degree 2 poles (-28.2482, 14.0469) (-28.2482, 14.2532) (-28.3682, 14.5211) (-28.476, 14.5981) knots 0 0 0 1 2 2 2
  spline S15 degree 2 poles (-28.476, 14.5981) (-28.5838, 14.6751) (-28.8764, 14.7336) (-29.0488, 14.7336) knots 0 0 0 1 2 2 2
  line L43 (-29.0488, 14.7336) -> (-29.2644, 14.7336)
  line L44 (-29.2644, 14.7336) -> (-29.2644, 15.1555)
  line L45 (-29.2644, 15.1555) -> (-29.095, 15.1555)
  spline S16 degree 2 poles (-29.095, 15.1555) (-28.7532, 15.1555) (-28.3221, 15.4819) (-28.3221, 15.7929) knots 0 0 0 1 2 2 2
  spline S17 degree 2 poles (-28.3221, 15.7929) (-28.3221, 15.9376) (-28.4329, 16.144) (-28.5222, 16.2056) knots 0 0 0 1 2 2 2
  spline S18 degree 2 poles (-28.5222, 16.2056) (-28.6177, 16.2702) (-28.8517, 16.3226) (-28.9841, 16.3226) knots 0 0 0 1 2 2 2
  line L46 (-22.6621, 16.6829) -> (-23.9708, 12.8829)
  line L47 (-23.9708, 12.8829) -> (-24.5159, 12.8829)
  line L48 (-24.5159, 12.8829) -> (-25.8247, 16.6829)
  line L49 (-25.8247, 16.6829) -> (-25.2827, 16.6829)
  line L50 (-25.2827, 16.6829) -> (-24.2295, 13.5265)
  line L51 (-24.2295, 13.5265) -> (-23.1764, 16.6829)
  line L52 (-23.1764, 16.6829) -> (-22.6621, 16.6829)
  line L53 (-16.7989, 12.8829) -> (-19.1423, 12.8829)
  line L54 (-19.1423, 12.8829) -> (-19.1423, 13.4218)
  spline S19 degree 2 poles (-19.1423, 13.4218) (-18.8898, 13.6589) (-18.4402, 14.0992) (-18.2247, 14.3363) knots 0 0 0 1 2 2 2
  spline S20 degree 2 poles (-18.2247, 14.3363) (-17.7905, 14.8137) (-17.4733, 15.3864) (-17.4733, 15.6913) knots 0 0 0 1 2 2 2
  spline S21 degree 2 poles (-17.4733, 15.6913) (-17.4733, 15.8514) (-17.5718, 16.0916) (-17.6611, 16.1686) knots 0 0 0 1 2 2 2
  spline S22 degree 2 poles (-17.6611, 16.1686) (-17.7504, 16.2456) (-17.9845, 16.3226) (-18.1261, 16.3226) knots 0 0 0 1 2 2 2
  spline S23 degree 2 poles (-18.1261, 16.3226) (-18.2616, 16.3226) (-18.5388, 16.2548) (-18.665, 16.2025) knots 0 0 0 1 2 2 2
  spline S24 degree 2 poles (-18.665, 16.2025) (-18.7728, 16.1594) (-18.973, 16.0362) (-19.0345, 15.9931) knots 0 0 0 1 2 2 2
  line L55 (-19.0345, 15.9931) -> (-19.0623, 15.9931)
  line L56 (-19.0623, 15.9931) -> (-19.0623, 16.5351)
  spline S25 degree 2 poles (-19.0623, 16.5351) (-18.9052, 16.612) (-18.3417, 16.7629) (-18.0892, 16.7629) knots 0 0 0 1 2 2 2
  spline S26 degree 2 poles (-18.0892, 16.7629) (-17.5564, 16.7629) (-16.9559, 16.1994) (-16.9559, 15.719) knots 0 0 0 1 2 2 2
  spline S27 degree 2 poles (-16.9559, 15.719) (-16.9559, 15.4942) (-17.0606, 15.1185) (-17.153, 14.9584) knots 0 0 0 1 2 2 2
  spline S28 degree 2 poles (-17.153, 14.9584) (-17.2454, 14.7921) (-17.5133, 14.4657) (-17.6611, 14.3086) knots 0 0 0 1 2 2 2
  spline S29 degree 2 poles (-17.6611, 14.3086) (-17.9013, 14.0469) (-18.4895, 13.4864) (-18.665, 13.3232) knots 0 0 0 1 2 2 2
  line L57 (-18.665, 13.3232) -> (-16.7989, 13.3232)
  line L58 (-16.7989, 13.3232) -> (-16.7989, 12.8829)
  line L59 (-11.7948, 16.6829) -> (-13.1036, 12.8829)
  line L60 (-13.1036, 12.8829) -> (-13.6486, 12.8829)
  line L61 (-13.6486, 12.8829) -> (-14.9574, 16.6829)
  line L62 (-14.9574, 16.6829) -> (-14.4154, 16.6829)
  line L63 (-14.4154, 16.6829) -> (-13.3623, 13.5265)
  line L64 (-13.3623, 13.5265) -> (-12.3091, 16.6829)
  line L65 (-12.3091, 16.6829) -> (-11.7948, 16.6829)
  line L66 (-6.1225, 12.8829) -> (-7.9764, 12.8829)
  line L67 (-7.9764, 12.8829) -> (-7.9764, 13.2709)
  line L68 (-7.9764, 13.2709) -> (-7.2866, 13.2709)
  line L69 (-7.2866, 13.2709) -> (-7.2866, 15.8175)
  line L70 (-7.2866, 15.8175) -> (-7.9764, 15.8175)
  line L71 (-7.9764, 15.8175) -> (-7.9764, 16.1655)
  spline S30 degree 2 poles (-7.9764, 16.1655) (-7.5853, 16.1655) (-7.2157, 16.3872) (-7.1911, 16.6952) knots 0 0 0 1 2 2 2
  line L72 (-7.1911, 16.6952) -> (-6.7969, 16.6952)
  line L73 (-6.7969, 16.6952) -> (-6.7969, 13.2709)
  line L74 (-6.7969, 13.2709) -> (-6.1225, 13.2709)
  line L75 (-6.1225, 13.2709) -> (-6.1225, 12.8829)
  line L76 (-0.9276, 16.6829) -> (-2.2363, 12.8829)
  line L77 (-2.2363, 12.8829) -> (-2.7814, 12.8829)
  line L78 (-2.7814, 12.8829) -> (-4.0901, 16.6829)
  line L79 (-4.0901, 16.6829) -> (-3.5482, 16.6829)
  line L80 (-3.5482, 16.6829) -> (-2.495, 13.5265)
  line L81 (-2.495, 13.5265) -> (-1.4418, 16.6829)
  line L82 (-1.4418, 16.6829) -> (-0.9276, 16.6829)
  line L83 (10.6761, 16.9864) -> (9.1607, 12.5864)
  line L84 (9.1607, 12.5864) -> (8.5296, 12.5864)
  line L85 (8.5296, 12.5864) -> (7.0142, 16.9864)
  line L86 (7.0142, 16.9864) -> (7.6418, 16.9864)
  line L87 (7.6418, 16.9864) -> (8.8612, 13.3316)
  line L88 (8.8612, 13.3316) -> (10.0807, 16.9864)
  line L89 (10.0807, 16.9864) -> (10.6761, 16.9864)
  spline S31 degree 2 poles (14.8301, 12.5009) (14.363, 12.5009) (13.5893, 12.7861) (13.3111, 13.0749) knots 0 0 0 1 2 2 2
  spline S32 degree 2 poles (13.3111, 13.0749) (13.033, 13.3673) (12.7371, 14.2302) (12.7371, 14.79) knots 0 0 0 1 2 2 2
  spline S33 degree 2 poles (12.7371, 14.79) (12.7371, 15.3213) (13.0366, 16.1628) (13.3147, 16.4623) knots 0 0 0 1 2 2 2
  spline S34 degree 2 poles (13.3147, 16.4623) (13.5821, 16.7511) (14.3666, 17.0649) (14.8337, 17.0649) knots 0 0 0 1 2 2 2
  spline S35 degree 2 poles (14.8337, 17.0649) (15.0583, 17.0649) (15.4648, 17.0007) (15.6502, 16.9436) knots 0 0 0 1 2 2 2
  spline S36 degree 2 poles (15.6502, 16.9436) (15.8, 16.9009) (16.1636, 16.744) (16.2742, 16.6869) knots 0 0 0 1 2 2 2
  line L90 (16.2742, 16.6869) -> (16.2742, 15.9809)
  line L91 (16.2742, 15.9809) -> (16.2243, 15.9809)
  spline S37 degree 2 poles (16.2243, 15.9809) (16.1137, 16.0772) (15.882, 16.2519) (15.668, 16.3517) knots 0 0 0 1 2 2 2
  spline S38 degree 2 poles (15.668, 16.3517) (15.4897, 16.4409) (15.0298, 16.5586) (14.7659, 16.5586) knots 0 0 0 1 2 2 2
  spline S39 degree 2 poles (14.7659, 16.5586) (14.1312, 16.5586) (13.3468, 15.603) (13.3468, 14.8078) knots 0 0 0 1 2 2 2
  spline S40 degree 2 poles (13.3468, 14.8078) (13.3468, 14.3657) (13.5536, 13.7025) (13.7497, 13.4743) knots 0 0 0 1 2 2 2
  spline S41 degree 2 poles (13.7497, 13.4743) (13.9387, 13.2461) (14.4735, 13.0072) (14.8087, 13.0072) knots 0 0 0 1 2 2 2
  spline S42 degree 2 poles (14.8087, 13.0072) (15.0547, 13.0072) (15.5468, 13.0785) (15.7144, 13.1498) knots 0 0 0 1 2 2 2
  line L92 (15.7144, 13.1498) -> (15.7144, 14.2872)
  line L93 (15.7144, 14.2872) -> (14.6946, 14.2872)
  line L94 (14.6946, 14.2872) -> (14.6946, 14.8007)
  line L95 (14.6946, 14.8007) -> (16.292, 14.8007)
  line L96 (16.292, 14.8007) -> (16.292, 12.8788)
  spline S43 degree 2 poles (16.292, 12.8788) (16.1815, 12.8289) (15.8035, 12.6756) (15.6431, 12.6292) knots 0 0 0 1 2 2 2
  spline S44 degree 2 poles (15.6431, 12.6292) (15.4256, 12.565) (15.0761, 12.5009) (14.8301, 12.5009) knots 0 0 0 1 2 2 2
  point P0 (0, 0)
  point P1 (-51.35, 14.7829)
  dimension "d88" = 10
  dimension "d89" = 10
  dimension "d90" = 0
  dimension "d91" = 0
  dimension "d92" = 0
  dimension "d93" = 0
  dimension "d94" = 4
  dimension "d95" = 6
  constraints: 1 midpoint, 4 other
  measures "d88" distance from line of point (-51.35, 14.783) L0
  measures "d89" distance between parallel lines of L10 L4
  measures "d90" distance between parallel lines of L9 L13
  measures "d91" distance between parallel lines of L11 L15
  measures "d92" distance between parallel lines of L8 L14
  measures "d93" distance between parallel lines of L6 L16
  measures "d94" distance between parallel lines of L1 L11
  measures "d95" distance between parallel lines of L11 L9
extrude "Extrusion8" cut sketch "Skizze14" against normal blind 1 contours L17 L18 L19 L20 L21 L22 L23 L24 L25 L26 L27 | L31 L32 L33 L34 L35 L36 L37 | S0 S1 L38 L39 S2 S3 S4 S5 L40 S6 S7 S8 S9 S10 L41 L42 S11 S12 S13 S14 S15 L43 L44 L45 S16 S17 S18 | L46 L47 L48 L49 L50 L51 L52 | L53 L54 S19 S20 S21 S22 S23 S24 L55 L56 S25 S26 S27 S28 S29 L57 L58 | L59 L60 L61 L62 L63 L64 L65 | L66 L67 L68 L69 L70 L71 S30 L72 L73 L74 L75 | L76 L77 L78 L79 L80 L81 L82 | L83 L84 L85 L86 L87 L88 L89 | S31 S32 S33 S34 S35 S36 L90 L91 S37 S38 S39 S40 S41 S42 L92 L93 L94 L95 L96 S43 S44
equation "\"d1\" = d0"
equation "\"d2\" = d0"
equation "\"d3\" = d0"
equation "\"d16\" = d15"
equation "\"d39\" = d36"
equation "\"d40\" = d36"
equation "\"d52\" = 0.5 * d51"
equation "\"d53\" = d52"
equation "\"d55\" = d54"
equation "\"d72\" = d71"
equation "\"d82\" = d81"
equation "\"d89\" = d88"
